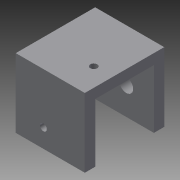
# Autodesk Inventor part: Corner
Saved by Autodesk Inventor 2015 SP1 (Build 190203100, 203)
## iProperties
Created: 2015-08-25
Part Number: Corner
Material: Generic
Document SubType Name: Modeling
Designer: Kartikye
Density: 1 g/cm^3
Appearance: Default
Author: Kartikye
Autodesk Inventor part; units mm, degrees
ref_plane "YZ Plane" through (0, 0, 0) normal (1, 0, 0) x (0, 1, 0)
ref_plane "XZ Plane" through (0, 0, 0) normal (0, 1, 0) x (-1, 0, 0)
ref_plane "XY Plane" through (0, 0, 0) normal (0, 0, 1) x (1, 0, 0)
sketch "Sketch1" plane through (0, 0, 0) normal (0, 1, 0) x (-1, 0, 0)
  line L0 (-5, 5) -> (5, 5)
  line L1 (5, 5) -> (5, -5)
  line L2 (5, -5) -> (-5, -5)
  line L3 (-5, -5) -> (-5, 5)
  line L4 (-5, 5) -> (5, -5) construction
  line L5 (5, 5) -> (-5, -5) construction
  point P0 (0, 0)
  dimension "d0" = 10
  dimension "d1" = 10
  constraints: 12 end point, 2 midpoint, 2 parallel, 1 horizontal, 1 perpendicular
  measures "d0" distance of L0.start L0.end
  measures "d1" distance of L0.end L1.end
extrude "Extrusion1" add sketch "Sketch1" along normal blind 1.5
sketch "Sketch3" plane through (0, 1.5, 0) normal (0, 1, 0) x (1, 0, 0)
  line L0 (-5, -5) -> (-5, 5)
  line L1 (-5, 5) -> (-3.5, 5)
  line L2 (5, 5) -> (-5, 5) projected
  line L3 (-3.5, 5) -> (-3.5, -3.5)
  line L4 (-3.5, -3.5) -> (5, -3.5)
  line L5 (5, -3.5) -> (5, -5)
  line L6 (5, -5) -> (-5, -5)
  point P0 (0, 0)
  dimension "d7" = 1.5
  dimension "d8" = 8.5
  dimension "d9" = 90
  constraints: 12 end point, 3 perpendicular, 1 point on line, 1 vertical
  measures "d7" distance of L0.end L1.end
  measures "d8" distance of L1.end L3.end
  measures "d9" angle of L1 L3
extrude "Extrusion2" add sketch "Sketch3" along normal blind 8.5
sketch "Sketch5" plane through (0, 1.5, 0) normal (0, 1, 0) x (1, 0, 0)
  circle A0 centre (-1, 2.3) radius 0.5
  line L0 (-3.5, 5) -> (-3.5, -3.5) projected
  line L1 (-3.5, -3.5) -> (5, -3.5) projected
  point P0 (0, 0)
  dimension "d14" = 1
  dimension "d15" = 2.5
  dimension "d16" = 5.8
  constraints: 1 centre point
  measures "d14" diameter of A0
  measures "d15" distance from line of A0.centre L0
  measures "d16" distance from line of L1 A0.centre
extrude "Extrusion4" cut sketch "Sketch5" against normal blind 8.5
sketch "Sketch6" plane through (-3.5, 1.5, 3.5) normal (1, 0, 0) x (0, 0, -1)
  circle A0 centre (2.5, 5.8) radius 0.5
  line L0 (8.5, 0) -> (0, 0) projected
  line L1 (0, 0) -> (0, 8.5) projected
  point P0 (3.5, -1.5)
  point P1 (0, 7)
  dimension "d19" = 1
  dimension "d20" = 5.8
  dimension "d21" = 2.5
  constraints: 1 centre point
  measures "d19" diameter of A0
  measures "d20" distance from line of L0 A0.centre
  measures "d21" distance from line of L1 A0.centre
extrude "Extrusion5" cut sketch "Sketch6" against normal blind 8.5
sketch "Sketch7" plane through (5, 1.5, 3.5) normal (0, 0, -1) x (-1, 0, 0)
  circle A0 centre (2.7, 2.5) radius 0.5
  line L0 (8.5, 0) -> (0, 0) projected
  line L1 (8.5, 0) -> (8.5, 8.5) projected
  point P0 (5, -1.5)
  dimension "d24" = 1
  dimension "d25" = 2.5
  dimension "d26" = 5.8
  constraints: 1 centre point
  measures "d24" diameter of A0
  measures "d25" distance from line of L0 A0.centre
  measures "d26" distance from line of L1 A0.centre
extrude "Extrusion6" cut sketch "Sketch7" against normal blind 8.5
sketch "Sketch8" plane through (0, 10, 0) normal (0, 1, 0) x (1, 0, 0)
  line L0 (5, -5) -> (5, 5)
  line L1 (5, 5) -> (-5, 5)
  line L2 (-5, 5) -> (-5, -5)
  line L3 (-5, -5) -> (5, -5)
  point P0 (0, 0)
  constraints: 8 end point, 3 perpendicular, 1 vertical
extrude "Extrusion7" add sketch "Sketch8" along normal blind 1.5
sketch "Sketch9" plane through (0, 11.5, 0) normal (0, 1, 0) x (1, 0, 0)
  circle A0 centre (1, 1) radius 1
  line L0 (-5, 5) -> (-5, -5) projected
  line L1 (-5, -5) -> (5, -5) projected
  point P0 (0, 0)
  dimension "d31" = 2
  dimension "d32" = 6
  dimension "d33" = 6
  constraints: 1 centre point
  measures "d31" diameter of A0
  measures "d32" distance from line of L0 A0.centre
  measures "d33" distance from line of A0.centre L1
extrude "Extrusion8" cut sketch "Sketch9" against normal blind 1.5
body "Solid1"
